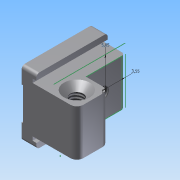
# Autodesk Inventor part: 4. Leiterplattenhalter_Links
Saved by Autodesk Inventor 2011 SP1 (Build 150282100, 282)
## iProperties
Created: 2012-05-07
Part Number: 4. Leiterplattenhalter_Links
Document SubType Name: Modeling
Designer: pburkhar
Density: 1 g/cm^3
Author: pburkhar
Autodesk Inventor part; units mm, degrees
ref_plane "YZ Plane" through (0, 0, 0) normal (1, 0, 0) x (0, 1, 0)
ref_plane "XZ Plane" through (0, 0, 0) normal (0, 1, 0) x (-1, 0, 0)
ref_plane "XY Plane" through (0, 0, 0) normal (0, 0, 1) x (1, 0, 0)
sketch "Skizze1" plane through (0, 0, 0) normal (0, 0, 1) x (1, 0, 0)
  line L0 (2.7, 9.6) -> (2.7, 4)
  arc A0 (2.7, 9.6) -> (2.2, 10.1) centre (2.2, 9.6) ccw
  line L1 (-0.6, 10.1) -> (2.2, 10.1)
  line L2 (-2.3, 10.1) -> (-0.6, 10.1)
  line L3 (-2.3, 10.1) -> (-2.3, 9.1)
  line L4 (-2.3, 9.1) -> (-2.3, 0)
  line L5 (-2.3, 0) -> (-2.3, -1)
  line L6 (-0.6, -1) -> (-2.3, -1)
  line L7 (-0.6, -0.995) -> (0, -0.995)
  line L8 (5.3, -1) -> (-0.6, -1)
  arc A1 (5.3, -1) -> (6.3, 0) centre (5.3, 0) ccw
  line L9 (6.3, 3) -> (6.3, 0)
  arc A2 (6.3, 3) -> (5.3, 4) centre (5.3, 3) ccw
  line L10 (2.7, 4) -> (5.3, 4)
  point P0 (0, 0)
  constraints: 22 end point, 6 point on circle, 3 centre point
extrude "Extrusion1" add sketch "Skizze1" along normal blind 10.2
sketch "Skizze2" plane through (-2.3, 10.1, 0) normal (0, 1, 0) x (1, 0, 0)
  line L0 (0, -10.2) -> (4.5, -10.2) projected
  line L1 (0, 0) -> (0, -10.2) projected
  line L2 (2.3, 0) -> (2.3, -0.9)
  line L3 (2.3, -0.9) -> (1.7, -0.9)
  line L4 (1.7, -0.9) -> (1.7, -1.5)
  line L5 (1.7, -1.5) -> (8.6, -1.5)
  line L6 (8.6, 0) -> (8.6, -10.2) projected
  line L7 (2.3, -10.2) -> (2.3, -9.3)
  line L8 (2.3, -9.3) -> (1.7, -9.3)
  line L9 (1.7, -9.3) -> (1.7, -8.7)
  line L10 (1.7, -8.7) -> (8.6, -8.7)
  line L11 (8.6, -1.5) -> (8.6, 0)
  line L12 (2.3, 0) -> (8.6, 0)
  line L13 (2.3, -10.2) -> (8.6, -10.2)
  line L14 (8.6, -8.7) -> (8.6, -10.2)
  dimension "d2" = 0.9
  dimension "d3" = 0.6
  dimension "d4" = 0.9
  dimension "d5" = 0.6
  dimension "d6" = 2.3
  dimension "d7" = 2.3
  dimension "d8" = 1.7
  dimension "d9" = 0.6
  dimension "d10" = 1.7
  constraints: 24 end point, 6 horizontal, 5 vertical, 3 point on line
  measures "d2" distance of L2.start L2.end
  measures "d3" distance of L3.end L4.end
  measures "d4" distance of L7.start L7.end
  measures "d5" distance of L8.end L9.end
  measures "d6" distance between parallel lines of L1 L7
  measures "d7" distance between parallel lines of L1 L2
  measures "d8" distance between parallel lines of L1 L4
  measures "d9" distance of L7.end L8.end
  measures "d10" distance between parallel lines of L1 L9
extrude "Extrusion2" cut sketch "Skizze2" against normal blind 12
sketch "Skizze3" plane through (2.7, 4, 8.7) normal (1, 0, 0) x (0, 0, -1)
  line L0 (0, 5.6) -> (0, 0) projected
  line L1 (7.2, 0) -> (0, 0) projected
  line L2 (7.2, 0) -> (7.2, 5.6) projected
  line L3 (7.2, 5.6) -> (0, 5.6) projected
  line L4 (7.2, 6.1) -> (0, 6.1) projected
  line L5 (-1.5, -5) -> (-1.5, 6.1) projected
  point P0 (8.7, -4)
  point P1 (3.55, 2.55)
  dimension "d13" = 3.55
  dimension "d14" = 5.05
  measures "d13" distance from line of L4 point (3.55, 2.55)
  measures "d14" distance from line of L5 point (3.55, 2.55)
sketch "Skizze4" plane through (-2.3, -1, 0) normal (-1, 0, 0) x (0, 0, 1)
  line L0 (10.2, 0) -> (10.2, 11.1) projected
  line L1 (0, 11.1) -> (10.2, 11.1) projected
  line L2 (0, 0) -> (0, 11.1) projected
  line L3 (10.2, 11.1) -> (10.2, 0) projected
  line L4 (10.2, 0) -> (0, 0) projected
  line L5 (0, 0) -> (0, 11.1) projected
  line L6 (0, 11.1) -> (10.2, 11.1) projected
  line L7 (10.2, 11.1) -> (10.2, 0) projected
  line L8 (10.2, 0) -> (0, 0) projected
  line L9 (0, 0) -> (0, 11.1) projected
  line L10 (0, 11.1) -> (10.2, 11.1) projected
  line L11 (10.2, 0) -> (10.2, 11.1) projected
  line L12 (0, 11.1) -> (10.2, 11.1) projected
  line L13 (0, 0) -> (0, 11.1) projected
  line L14 (0, 0) -> (10.2, 0) projected
  line L15 (8.7, 10.6) -> (8.7, 5) projected
  line L16 (1.5, 5) -> (8.7, 5) projected
  line L17 (1.5, 5) -> (1.5, 10.6) projected
  line L18 (1.5, 10.6) -> (8.7, 10.6) projected
  point P0 (0, 1)
  point P1 (5.1, 7.55)
  dimension "d15" = 3.55
  dimension "d16" = 5.1
  dimension "d17" = 5.1
  measures "d15" distance from line of L1 point (5.1, 7.55)
  measures "d16" distance from line of L0 point (5.1, 7.55)
  measures "d17" distance from line of L2 point (5.1, 7.55)
hole "Hole1" at (-2.3, 6.55, 5.1) direction (1, 0, 0) diameter 2.013 end through all countersink diameter 4 countersink angle 90 thread size "M2.5x0.45" class "6H" standard "ANSI Metric M Profile"
sketch "Skizze5" plane through (2.2, 10.1, 1.5) normal (0, 0, -1) x (-1, 0, 0)
  line L0 (-4.1, -10.1) -> (-4.1, -7.1) projected
  line L1 (2.8, -11.1) -> (-3.1, -11.1) projected
  line L2 (-3.1, -6.1) -> (-0.5, -6.1) projected
  line L3 (2.2, 0) -> (2.2, -11.1) projected
  point P0 (2.2, -10.1)
  point P1 (-1.6, -8.6)
  dimension "d25" = 2.5
  dimension "d26" = 2.5
  dimension "d27" = 2.5
  dimension "d28" = 3.8
  measures "d25" distance from line of L2 point (-1.6, -8.6)
  measures "d26" distance from line of L0 point (-1.6, -8.6)
  measures "d27" distance from line of L1 point (-1.6, -8.6)
  measures "d28" distance from line of L3 point (-1.6, -8.6)
sketch "Skizze6" plane through (-0.6, 10.1, 8.7) normal (0, 0, 1) x (1, 0, 0)
  line L0 (6.9, -7.1) -> (6.9, -10.1) projected
  line L1 (3.3, -6.1) -> (5.9, -6.1) projected
  line L2 (0.6, -11.1) -> (0.6, 0) projected
  point P0 (0.6, -10.1)
  point P1 (4.4, -8.6)
  dimension "d29" = 2.5
  dimension "d30" = 2.5
  dimension "d31" = 3.8
  measures "d29" distance from line of L1 point (4.4, -8.6)
  measures "d30" distance from line of L0 point (4.4, -8.6)
  measures "d31" distance from line of L2 point (4.4, -8.6)
hole "Hole2" at (3.8, 1.5, 8.7) direction (0, 0, -1) diameter 2.013 depth 6 tip angle 118 countersink diameter 4 countersink angle 90 thread size "M2.5x0.45" class "6H" standard "ANSI Metric M Profile"
hole "Hole3" at (3.8, 1.5, 1.5) direction (0, 0, 1) diameter 2.013 depth 6 tip angle 118 countersink diameter 4 countersink angle 90 thread size "M2.5x0.45" class "6H" standard "ANSI Metric M Profile"
sketch "Skizze7" plane through (-2.3, 10.1, 10.2) normal (0, 1, 0) x (1, 0, 0)
  line L0 (0, 10.2) -> (2.3, 10.2) projected
  line L1 (0, 10.2) -> (0, 0) projected
  line L2 (0, 0) -> (2.3, 0) projected
  line L3 (0, 7.65) -> (0.2, 7.65)
  line L4 (0.2, 7.65) -> (0.2, 2.55)
  line L5 (0.2, 2.55) -> (0, 2.55)
  line L6 (0, 7.65) -> (0, 2.55)
  dimension "d46" = 2.55
  dimension "d47" = 2.55
  dimension "d48" = 0.2
  constraints: 8 end point, 2 horizontal, 2 point on line, 2 vertical
  measures "d46" distance between parallel lines of L0 L3
  measures "d47" distance between parallel lines of L2 L5
  measures "d48" distance between parallel lines of L1 L4
extrude "Extrusion3" cut sketch "Skizze7" against normal blind 12
fillet "Rundung1" radius 0.5 1 edges at (-1.15, 10.1, 10.2)
fillet "Rundung2" radius 0.5 3 edges at (-1.15, 10.1, 0) (-1.15, -1, 0) (-1.15, -1, 10.2)
